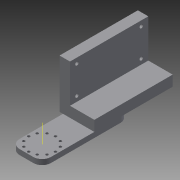
# Autodesk Inventor part: first_man_link
Saved by Autodesk Inventor 2015 (Build 190159000, 159)
## iProperties
Created: 2014-10-20
Part Number: first_man_link
Material: Generic
Document SubType Name: Modeling
Designer: ericd_000
Density: 1 g/cm^3
Appearance: Default
Author: ericd_000
Autodesk Inventor part; units mm, degrees
ref_plane "YZ Plane" through (0, 0, 0) normal (1, 0, 0) x (0, 1, 0)
ref_plane "XZ Plane" through (0, 0, 0) normal (0, 1, 0) x (-1, 0, 0)
ref_plane "XY Plane" through (0, 0, 0) normal (0, 0, 1) x (1, 0, 0)
sketch "Sketch1" plane through (0, 0, 0) normal (0, 0, 1) x (1, 0, 0)
  line L0 (-9, 25) -> (9, 25)
  line L1 (9, 25) -> (9, -25)
  line L2 (9, -25) -> (-9, -25)
  line L3 (-9, -25) -> (-9, 25)
  point P0 (0, 0)
  point P1 (0, 25)
  point P2 (-9, 0)
  dimension "d0" = 18
  dimension "d1" = 50
  constraints: 8 end point, 2 midpoint, 2 parallel, 1 horizontal, 1 horizontal alignment, 1 perpendicular, 1 vertical alignment
  measures "d0" distance of L1.end L2.end
  measures "d1" distance of L0.end L1.end
extrude "Extrusion1" add sketch "Sketch1" along normal blind 3
fillet "Fillet1" radius 5 2 edges at (-9, -25, 1.5) (9, -25, 1.5)
fillet "Fillet2" radius 5 2 edges at (-9, 25, 1.5) (9, 25, 1.5)
sketch "Sketch2" plane through (0, 0, 3) normal (0, 0, 1) x (1, 0, 0)
  circle A0 centre (0, -16) radius 9
  circle A1 centre (0, 16) radius 9
  line L0 (-4, -25) -> (4, -25) projected
  circle A2 centre (0, -8.304) radius 0.75
  line L1 (4, 25) -> (-4, 25) projected
  point P0 (0, 0)
  dimension "d6" = 18
  dimension "d8" = 1.5
  dimension "d10" = 18
  constraints: 3 centre point, 2 tangent
  measures "d6" diameter of A0
  measures "d8" diameter of A2
  measures "d10" diameter of A1
extrude "Extrusion2" cut sketch "Sketch2" against normal up to surface (3 mm away) contours A2
pattern_circular "Circular Pattern1" count 12 over 360 about axis through (0, -16, 3) along (0, 0, 1) of "Extrusion2"
sketch "Sketch4" plane through (0, 0, 3) normal (0, 0, 1) x (1, 0, 0)
  line L0 (-11, 5) -> (9, 5)
  line L1 (9, 5) -> (9, 50)
  line L2 (9, 50) -> (-11, 50)
  line L3 (-11, 50) -> (-11, 5)
  line L4 (-9, 20) -> (-9, -20) projected
  line L5 (4, 25) -> (-4, 25) projected
  line L6 (9, -20) -> (9, 20) projected
  point P0 (0, 0)
  dimension "d25" = 20
  dimension "d26" = 45
  dimension "d27" = 20
  constraints: 8 end point, 2 parallel, 1 collinear, 1 horizontal, 1 perpendicular
  measures "d25" distance of L1.end L2.end
  measures "d26" distance of L2.end L0.start
  measures "d27" distance between parallel lines of L5 L0
extrude "Extrusion5" add sketch "Sketch4" along normal blind 6
sketch "Sketch5" plane through (0, 0, 3) normal (0, 0, 1) x (1, 0, 0)
  line L0 (9, 50) -> (-11, 50) projected
  line L1 (-5, 5) -> (-11, 5)
  line L2 (-11, 5) -> (-11, 50)
  line L3 (-11, 50) -> (-5, 50)
  line L4 (-5, 50) -> (-5, 5)
  line L5 (-11, 50) -> (-11, 5) projected
  point P0 (0, 0)
  dimension "d30" = 6
  constraints: 8 end point, 2 parallel, 1 collinear, 1 horizontal, 1 perpendicular, 1 point on line
  measures "d30" distance between parallel lines of L4 L2
extrude "Extrusion6" add sketch "Sketch5" along normal blind 28
sketch "Sketch6" plane through (-11, 5, 3) normal (-1, 0, 0) x (0, 0, 1)
  circle A0 centre (25, 4) radius 1
  circle A1 centre (9, 4) radius 1
  circle A2 centre (25, 41) radius 1
  circle A3 centre (9, 41) radius 1
  line L0 (0, 0) -> (28, 0) projected
  line L1 (25, 4) -> (25, 41) construction
  line L2 (28, 45) -> (28, 0) projected
  point P0 (-3, -5)
  point P1 (28, 22.5)
  point P2 (25, 22.5)
  point P3 (6, 0)
  dimension "d33" = 2
  dimension "d34" = 2
  dimension "d35" = 2
  dimension "d36" = 2
  dimension "d37" = 37
  dimension "d38" = 16
  dimension "d40" = 16
  dimension "d43" = 3
  constraints: 4 centre point, 3 horizontal alignment, 2 end point, 2 midpoint, 1 vertical alignment
  measures "d33" diameter of A0
  measures "d34" diameter of A1
  measures "d35" diameter of A2
  measures "d36" diameter of A3
  measures "d37" distance of L1.end L1.start
  measures "d38" distance of A1.centre L1.start
  measures "d40" distance of A3.centre L1.end
  measures "d43" distance from line of L2 L1.end
extrude "Extrusion7" cut sketch "Sketch6" against normal up to surface (20 mm away)
body "Solid1"
